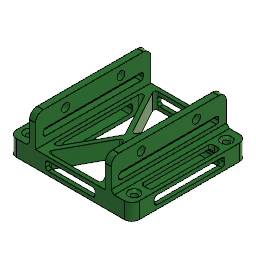
Full Motor Build (Goalie) (Autodesk Fusion 360 archive; units mm, degrees)
design "LGR Foundation"
Autodesk Fusion 360 part; units mm, degrees
(part 1 of 5)
sketch "Sketch1" plane through (0, 0, 0) normal (0, 0, 1) x (1, 0, 0)
  line L0 (-40, 37.5) -> (40, 37.5)
  line L1 (40, 37.5) -> (40, -37.5)
  line L2 (40, -37.5) -> (-40, -37.5)
  line L3 (-40, -37.5) -> (-40, 37.5)
  dimension "d1" = 80
  dimension "d2" = 75
  dimension "d3" = 37.5
  dimension "d4" = 40
  constraint horizontal L0
  constraint vertical L1
  constraint horizontal L2
  constraint vertical L3
  measures "d1" distance of L1 L3
  measures "d2" distance of L0 L2
  measures "d3" distance of origin L2
  measures "d4" distance of origin L1
extrude "Extrude1" add sketch "Sketch1" along normal blind 6
sketch "Sketch2" plane through (0, 0, 6) normal (0, 0, 1) x (-1, 0, 0)
  line L0 (40, 37.5) -> (-40, 37.5)
  line L1 (-40, 37.5) -> (-40, -37.5)
  line L2 (-40, -37.5) -> (40, -37.5)
  line L3 (40, -37.5) -> (40, 37.5)
  line L4 (26.55, -37.5) -> (22.55, -37.5)
  line L5 (22.55, -37.5) -> (22.55, 37.5)
  line L6 (22.55, 37.5) -> (26.55, 37.5)
  line L7 (26.55, 37.5) -> (26.55, -37.5)
  line L8 (-22.55, -37.5) -> (-26.55, -37.5)
  line L9 (-26.55, -37.5) -> (-26.55, 37.5)
  line L10 (-26.55, 37.5) -> (-22.55, 37.5)
  line L11 (-22.55, 37.5) -> (-22.55, -37.5)
  dimension "d7" = 45.1
  dimension "d8" = 53.1
  dimension "d9" = 13.45
  dimension "d10" = 17.45
  constraint horizontal L4
  constraint vertical L5
  constraint horizontal L6
  constraint vertical L7
  constraint coincident L0 L5.end
  constraint coincident L2 L4.start
  constraint horizontal L8
  constraint vertical L9
  constraint horizontal L10
  constraint vertical L11
  constraint coincident L0 L9.end
  constraint coincident L2 L8.start
  measures "d7" distance of L5 L11
  measures "d8" distance of L7 L9
  measures "d9" distance of L3 L7
  measures "d10" distance of L3 L5
extrude "Extrude2" add sketch "Sketch2" along normal blind 20 contours L0 L2 L4 L5 L6 L7 | L0 L2 L8 L9 L10 L11
sketch "Sketch3" plane through (26.55, 0, 0) normal (1, 0, 0) x (0, 1, 0)
  line L0 (-37.5, 6) -> (37.5, 6)
  line L1 (37.5, 6) -> (37.5, 26)
  line L2 (37.5, 26) -> (-37.5, 26)
  line L3 (-37.5, 26) -> (-37.5, 6)
  circle A0 centre (-18, 20) radius 2.55
  circle A1 centre (18, 20) radius 2.55
  line L4 (37.5, 0) -> (-37.5, 0)
  dimension "d13" = 5.1
  dimension "d14" = 5.1
  dimension "d15" = 20
  dimension "d16" = 36
  dimension "d17" = 19.5
  constraint horizontal A0.centre A1.centre
  measures "d13" diameter of A0
  measures "d14" diameter of A1
  measures "d15" distance of A0.centre L4
  measures "d16" distance of A0.centre A1.centre
  measures "d17" distance of L1 A1.centre
extrude "Extrude3" cut sketch "Sketch3" along normal blind 0 and the other way blind 53.1 contours A0 | A1
chamfer "Chamfer1" distance 2 angle 45 2 edges at (26.55, 0, 6) (-26.55, 0, 6)
sketch "Sketch8" plane through (0, 0, 6) normal (0, 0, 1) x (-1, 0, 0)
  line L0 (28.55, 37.5) -> (28.55, -37.5)
  line L1 (28.55, -37.5) -> (40, -37.5)
  line L2 (40, -37.5) -> (40, 37.5)
  line L3 (40, 37.5) -> (28.55, 37.5)
  line L4 (-40, 37.5) -> (-40, -37.5)
  line L5 (-40, -37.5) -> (-28.55, -37.5)
  point P0 (34, -30)
  point P1 (-34, -30)
  point P2 (-34, 30)
  point P3 (34, 30)
  dimension "d57" = 68
  dimension "d58" = 60
  dimension "d59" = 6
  dimension "d60" = 7.5
  constraint horizontal P0 P1
  constraint vertical P1 P2
  constraint horizontal P2 P3
  constraint vertical P0 P3
  measures "d57" distance of P0 P1
  measures "d58" distance of P1 P2
  measures "d59" distance of P1 L4
  measures "d60" distance of P1 L5
hole "Hole3" at (-34, 30, 6) at (-34, -30, 6) at (34, -30, 6) at (34, 30, 6) direction (0, 0, -1) diameter 3.797 end through all countersink diameter 7.087 countersink angle 100
fillet "Fillet1" radius 5 4 edges at (40, -37.5, 3) (40, 37.5, 3) (-40, -37.5, 3) (-40, 37.5, 3)
fillet "Fillet2" radius 5 4 edges at (24.55, -37.5, 26) (-24.55, -37.5, 26) (-24.55, 37.5, 26) (24.55, 37.5, 26)
sketch "Sketch13" plane through (0, 0, 6) normal (0, 0, 1) x (-1, 0, 0)
  line L0 (-22.55, 37.5) -> (-22.55, -37.5)
  line L1 (-22.55, -37.5) -> (22.55, -37.5)
  line L2 (22.55, -37.5) -> (22.55, 37.5)
  line L3 (22.55, 37.5) -> (-22.55, 37.5)
  line L4 (20.05, 27.1318) -> (20.05, -27.1318)
  line L5 (15.4698, 35) -> (-15.4698, 35)
  line L6 (-20.05, 27.1318) -> (-20.05, -27.1318)
  line L7 (15.4698, -35) -> (-15.4698, -35)
  line L8 (17.234, 27.8516) -> (2.3937, 0.7198)
  line L9 (2.3937, -0.7198) -> (17.234, -27.8516)
  line L10 (16.7858, -32.7802) -> (1.316, -4.4974)
  line L11 (-1.316, -4.4974) -> (-16.7858, -32.7802)
  line L12 (-17.234, -27.8516) -> (-2.3937, -0.7198)
  line L13 (-2.3937, 0.7198) -> (-17.234, 27.8516)
  line L14 (-16.7858, 32.7802) -> (-1.316, 4.4974)
  line L15 (1.316, 4.4974) -> (16.7858, 32.7802)
  arc A0 (20.05, 27.1318) -> (17.234, 27.8516) centre (18.55, 27.1318) ccw
  arc A1 (17.234, -27.8516) -> (20.05, -27.1318) centre (18.55, -27.1318) ccw
  arc A2 (15.4698, -35) -> (16.7858, -32.7802) centre (15.4698, -33.5) ccw
  arc A3 (16.7858, 32.7802) -> (15.4698, 35) centre (15.4698, 33.5) ccw
  arc A4 (-15.4698, 35) -> (-16.7858, 32.7802) centre (-15.4698, 33.5) ccw
  arc A5 (-17.234, 27.8516) -> (-20.05, 27.1318) centre (-18.55, 27.1318) ccw
  arc A6 (-20.05, -27.1318) -> (-17.234, -27.8516) centre (-18.55, -27.1318) ccw
  arc A7 (-16.7858, -32.7802) -> (-15.4698, -35) centre (-15.4698, -33.5) ccw
  arc A8 (1.316, -4.4974) -> (-1.316, -4.4974) centre (0, -5.2172) ccw
  arc A9 (2.3937, 0.7198) -> (2.3937, -0.7198) centre (3.7097, 0) ccw
  arc A10 (-1.316, 4.4974) -> (1.316, 4.4974) centre (0, 5.2172) ccw
  arc A11 (-2.3937, -0.7198) -> (-2.3937, 0.7198) centre (-3.7097, 0) ccw
  point P0 (20.05, 33)
  point P1 (20.05, -33)
  point P2 (18, 35)
  point P3 (-18, 35)
  point P4 (-20.05, 33)
  point P5 (-20.05, -33)
  point P6 (18, -35)
  point P7 (-18, -35)
  dimension "d91" = 2.5
  dimension "d92" = 2.5
  dimension "d93" = 66
  dimension "d95" = 66
  dimension "d96" = 2.5
  dimension "d97" = 36
  dimension "d98" = 36
  dimension "d99" = 2.5
  dimension "d100" = 4.55
  dimension "d101" = 4.55
  dimension "d102" = 4.5
  dimension "d103" = 4.5
  dimension "d104" = 1.5
  constraint vertical L4
  constraint horizontal L5
  constraint parallel L0 L6
  constraint horizontal L7
  constraint parallel L9 L10
  constraint parallel L8 L11
  constraint parallel L11 L12
  constraint parallel L13 L14
  constraint coincident P0 L4
  constraint coincident P0 L8
  constraint tangent L4 A0
  constraint tangent L8 A0
  constraint coincident P1 L4
  constraint coincident P1 L9
  constraint tangent L4 A1
  constraint tangent L9 A1
  constraint equal A0 A1
  constraint coincident P6 L10
  constraint coincident P6 L7
  constraint tangent L10 A2
  constraint tangent L7 A2
  constraint equal A0 A2
  constraint coincident P2 L15
  constraint coincident P2 L5
  constraint tangent L15 A3
  constraint tangent L5 A3
  constraint equal A0 A3
  constraint coincident P3 L14
  constraint coincident P3 L5
  constraint tangent L14 A4
  constraint tangent L5 A4
  constraint equal A0 A4
  constraint coincident P4 L13
  constraint coincident P4 L6
  constraint tangent L13 A5
  constraint tangent L6 A5
  constraint equal A0 A5
  constraint coincident P5 L6
  constraint coincident P5 L12
  constraint tangent L6 A6
  constraint tangent L12 A6
  constraint equal A0 A6
  constraint coincident P7 L11
  constraint coincident P7 L7
  constraint tangent L11 A7
  constraint tangent L7 A7
  constraint equal A0 A7
  constraint tangent L10 A8
  constraint tangent L11 A8
  constraint equal A0 A8
  constraint tangent L9 A9
  constraint tangent L8 A9
  constraint equal A0 A9
  constraint tangent L15 A10
  constraint tangent L14 A10
  constraint equal A0 A10
  constraint tangent L13 A11
  constraint tangent L12 A11
  constraint equal A0 A11
  measures "d91" distance of L2 L4
  measures "d92" distance of L3 L5
  measures "d93" distance of P0 P1
  measures "d95" distance of P4 P5
  measures "d96" distance of L0 L6
  measures "d97" distance of P6 P7
  measures "d98" distance of P2 P3
  measures "d99" distance of L1 L7
  measures "d100" distance of L2 P6
  measures "d101" distance of L2 P2
  measures "d102" distance of L3 P0
  measures "d103" distance of L3 P4
  measures "d104" radius of A0
extrude "Extrude6" cut sketch "Sketch13" along normal blind 0 and the other way blind 6 contours L4 L8 L9 A0 A1 A9 | L5 L14 L15 A3 A4 A10 | L6 L12 L13 A5 A6 A11 | L7 L10 L11 A2 A7 A8
extrude "Extrude7" cut 1 faces at (29.1614, 9.0439, 0) along direction (0, 0, -1) blind 0 and the other way blind 0.4
ref_plane "WorkPlane3" through (34.275, 0, 1.9) normal (0, 0, 1) x (1, 0, 0)
sketch "Sketch14" plane through (0, 0, 1.9) normal (0, 0, 1) x (1, 0, 0)
  circle A0 centre (34, 30) radius 4.5
  circle A1 centre (-34, 30) radius 4.5
  circle A2 centre (-34, -30) radius 4.5
  circle A3 centre (34, -30) radius 4.5
  line L0 (35, 37.5) -> (28.55, 37.5)
  line L1 (40, -32.5) -> (40, 32.5)
  dimension "d115" = 9
  dimension "d116" = 9
  dimension "d117" = 9
  dimension "d118" = 9
  dimension "d119" = 68
  dimension "d120" = 60
  dimension "d121" = 7.5
  dimension "d122" = 6
  constraint horizontal A0.centre A1.centre
  constraint vertical A0.centre A3.centre
  constraint horizontal A2.centre A3.centre
  constraint vertical A1.centre A2.centre
  measures "d115" diameter of A0
  measures "d116" diameter of A1
  measures "d117" diameter of A2
  measures "d118" diameter of A3
  measures "d119" distance of A0.centre A1.centre
  measures "d120" distance of A0.centre A3.centre
  measures "d121" distance of A0.centre L0
  measures "d122" distance of A0.centre L1
ref_plane "WorkPlane4" through (34.275, 0, 0.4) normal (0, 0, 1) x (1, 0, 0)
sketch "Sketch17" plane through (0, 0, 6) normal (0, 0, 1) x (-1, 0, 0)
  arc A0 (-40, -32.5) -> (-35, -37.5) centre (-35, -32.5) ccw
  line L0 (-35, -37.5) -> (-28.55, -37.5)
  line L1 (-28.55, -37.5) -> (-28.55, 37.5)
  line L2 (-28.55, 37.5) -> (-35, 37.5)
  arc A1 (-35, 37.5) -> (-40, 32.5) centre (-35, 32.5) ccw
  line L3 (-40, 32.5) -> (-40, -32.5)
  line L4 (-33.05, -23) -> (-35.5, -23)
  line L5 (-37.5, -21) -> (-37.5, 21)
  line L6 (-35.5, 23) -> (-33.05, 23)
  line L7 (-31.05, 21) -> (-31.05, -21)
  arc A2 (-33.05, -23) -> (-31.05, -21) centre (-33.05, -21) ccw
  arc A3 (-31.05, 21) -> (-33.05, 23) centre (-33.05, 21) ccw
  arc A4 (-35.5, 23) -> (-37.5, 21) centre (-35.5, 21) ccw
  arc A5 (-37.5, -21) -> (-35.5, -23) centre (-35.5, -21) ccw
  line L8 (35.5, -23) -> (33.05, -23)
  line L9 (31.05, -21) -> (31.05, 21)
  line L10 (33.05, 23) -> (35.5, 23)
  line L11 (37.5, 21) -> (37.5, -21)
  line L12 (28.55, -37.5) -> (28.55, 37.5)
  line L13 (40, -32.5) -> (40, 32.5)
  arc A6 (35.5, -23) -> (37.5, -21) centre (35.5, -21) ccw
  arc A7 (31.05, -21) -> (33.05, -23) centre (33.05, -21) ccw
  arc A8 (33.05, 23) -> (31.05, 21) centre (33.05, 21) ccw
  arc A9 (37.5, 21) -> (35.5, 23) centre (35.5, 21) ccw
  circle A10 centre (-34, 30) radius 3.5435
  circle A11 centre (-34, -30) radius 3.5435
  point P0 (-34, -30)
  point P1 (-34, 30)
  point P2 (34, -30)
  point P3 (34, 30)
  dimension "d134" = 2.5
  dimension "d135" = 2.5
  dimension "d136" = 7
  dimension "d137" = 7
  dimension "d138" = 2
  dimension "d141" = 2.5
  dimension "d142" = 2.5
  dimension "d143" = 7
  dimension "d144" = 7
  dimension "d145" = 2
  constraint horizontal L4
  constraint vertical L5
  constraint horizontal L6
  constraint vertical L7
  constraint tangent L4 A2
  constraint tangent L7 A2
  constraint tangent L6 A3
  constraint tangent L7 A3
  constraint equal A2 A3
  constraint tangent L6 A4
  constraint tangent L5 A4
  constraint equal A2 A4
  constraint tangent L5 A5
  constraint tangent L4 A5
  constraint equal A2 A5
  constraint horizontal L8
  constraint vertical L9
  constraint horizontal L10
  constraint vertical L11
  constraint tangent L8 A6
  constraint tangent L11 A6
  constraint tangent L9 A7
  constraint tangent L8 A7
  constraint equal A6 A7
  constraint tangent L9 A8
  constraint tangent L10 A8
  constraint equal A6 A8
  constraint tangent L10 A9
  constraint tangent L11 A9
  constraint equal A6 A9
  measures "d134" distance of L1 L7
  measures "d135" distance of L3 L5
  measures "d136" distance of L4 P0
  measures "d137" distance of L6 P1
  measures "d138" radius of A2
  measures "d141" distance of L9 L12
  measures "d142" distance of L11 L13
  measures "d143" distance of L8 P2
  measures "d144" distance of L10 P3
  measures "d145" radius of A6
extrude "Extrude10" cut sketch "Sketch17" against normal blind 5.6 contours L4 L5 L6 L7 A2 A3 A4 A5 | L8 L9 L10 L11 A6 A7 A8 A9
extrude "Extrude12" add 1 faces at (-23.7167, 7, 0.4) along direction (0, 0, -1) blind 5
sketch "Sketch18" plane through (0, -37.5, 0) normal (0, -1, 0) x (1, 0, 0)
  line L0 (35, -4.6) -> (35, 6)
  line L1 (35, 6) -> (28.55, 6)
  line L2 (28.55, 6) -> (26.55, 8)
  line L3 (26.55, 8) -> (26.55, 21)
  line L4 (26.55, 21) -> (22.55, 21)
  line L5 (22.55, 21) -> (22.55, 6)
  line L6 (22.55, 6) -> (-22.55, 6)
  line L7 (-22.55, 6) -> (-22.55, 21)
  line L8 (-22.55, 21) -> (-26.55, 21)
  line L9 (-26.55, 21) -> (-26.55, 8)
  line L10 (-26.55, 8) -> (-28.55, 6)
  line L11 (-28.55, 6) -> (-35, 6)
  line L12 (-35, 6) -> (-35, -4.6)
  line L13 (-35, -4.6) -> (35, -4.6)
  line L14 (-14.5, 3.5) -> (14.5, 3.5)
  line L15 (16, 2) -> (16, -0.6)
  line L16 (14.5, -2.1) -> (-14.5, -2.1)
  line L17 (-16, -0.6) -> (-16, 2)
  arc A0 (-14.5, 3.5) -> (-16, 2) centre (-14.5, 2) ccw
  arc A1 (-16, -0.6) -> (-14.5, -2.1) centre (-14.5, -0.6) ccw
  arc A2 (14.5, -2.1) -> (16, -0.6) centre (14.5, -0.6) ccw
  arc A3 (16, 2) -> (14.5, 3.5) centre (14.5, 2) ccw
  dimension "d154" = 32
  dimension "d155" = 2.5
  dimension "d156" = 2.5
  dimension "d157" = 16
  dimension "d158" = 1.5
  constraint horizontal L14
  constraint vertical L15
  constraint horizontal L16
  constraint vertical L17
  constraint tangent L14 A0
  constraint tangent L17 A0
  constraint tangent L17 A1
  constraint tangent L16 A1
  constraint equal A0 A1
  constraint tangent L16 A2
  constraint tangent L15 A2
  constraint equal A0 A2
  constraint tangent L15 A3
  constraint tangent L14 A3
  constraint equal A0 A3
  measures "d154" distance of L15 L17
  measures "d155" distance of L6 L14
  measures "d156" distance of L13 L16
  measures "d157" distance of origin L17
  measures "d158" radius of A0
extrude "Extrude13" cut sketch "Sketch18" against normal blind 4 contours L14 L15 L16 L17 A0 A1 A2 A3
sketch "Sketch19" plane through (0, 37.5, 0) normal (0, 1, 0) x (-1, 0, 0)
  line L0 (35, -4.6) -> (35, 6)
  line L1 (35, 6) -> (28.55, 6)
  line L2 (28.55, 6) -> (26.55, 8)
  line L3 (26.55, 8) -> (26.55, 21)
  line L4 (26.55, 21) -> (22.55, 21)
  line L5 (22.55, 21) -> (22.55, 6)
  line L6 (22.55, 6) -> (-22.55, 6)
  line L7 (-22.55, 6) -> (-22.55, 21)
  line L8 (-22.55, 21) -> (-26.55, 21)
  line L9 (-26.55, 21) -> (-26.55, 8)
  line L10 (-26.55, 8) -> (-28.55, 6)
  line L11 (-28.55, 6) -> (-35, 6)
  line L12 (-35, 6) -> (-35, -4.6)
  line L13 (-35, -4.6) -> (35, -4.6)
  line L14 (-14.5, 3.5) -> (14.5, 3.5)
  line L15 (16, 2) -> (16, -0.6)
  line L16 (14.5, -2.1) -> (-14.5, -2.1)
  line L17 (-16, -0.6) -> (-16, 2)
  arc A0 (-14.5, 3.5) -> (-16, 2) centre (-14.5, 2) ccw
  arc A1 (-16, -0.6) -> (-14.5, -2.1) centre (-14.5, -0.6) ccw
  arc A2 (14.5, -2.1) -> (16, -0.6) centre (14.5, -0.6) ccw
  arc A3 (16, 2) -> (14.5, 3.5) centre (14.5, 2) ccw
  dimension "d161" = 2.5
  dimension "d162" = 2.5
  dimension "d163" = 32
  dimension "d164" = 16
  dimension "d165" = 1.5
  constraint horizontal L14
  constraint vertical L15
  constraint horizontal L16
  constraint vertical L17
  constraint tangent L14 A0
  constraint tangent L17 A0
  constraint tangent L17 A1
  constraint tangent L16 A1
  constraint equal A0 A1
  constraint tangent L16 A2
  constraint tangent L15 A2
  constraint equal A0 A2
  constraint tangent L15 A3
  constraint tangent L14 A3
  constraint equal A0 A3
  measures "d161" distance of L13 L16
  measures "d162" distance of L6 L14
  measures "d163" distance of L15 L17
  measures "d164" distance of origin L17
  measures "d165" radius of A0
extrude "Extrude14" cut sketch "Sketch19" against normal blind 4 contours L14 L15 L16 L17 A0 A1 A2 A3
sketch "Sketch20" plane through (-40, 0, 0) normal (-1, 0, 0) x (0, -1, 0)
  line L0 (32.5, -4.6) -> (32.5, 6)
  line L1 (32.5, 6) -> (-32.5, 6)
  line L2 (-32.5, 6) -> (-32.5, -4.6)
  line L3 (-32.5, -4.6) -> (32.5, -4.6)
  line L4 (-21, 3.5) -> (21, 3.5)
  line L5 (23, 1.5) -> (23, -0.1)
  line L6 (21, -2.1) -> (-21, -2.1)
  line L7 (-23, -0.1) -> (-23, 1.5)
  line L8 (-32.5, 6) -> (32.5, 6)
  arc A0 (-21, 3.5) -> (-23, 1.5) centre (-21, 1.5) ccw
  arc A1 (-23, -0.1) -> (-21, -2.1) centre (-21, -0.1) ccw
  arc A2 (21, -2.1) -> (23, -0.1) centre (21, -0.1) ccw
  arc A3 (23, 1.5) -> (21, 3.5) centre (21, 1.5) ccw
  dimension "d168" = 2.5
  dimension "d169" = 2.5
  dimension "d170" = 46
  dimension "d171" = 23
  dimension "d172" = 2
  constraint horizontal L4
  constraint vertical L5
  constraint horizontal L6
  constraint vertical L7
  constraint tangent L4 A0
  constraint tangent L7 A0
  constraint tangent L7 A1
  constraint tangent L6 A1
  constraint equal A0 A1
  constraint tangent L6 A2
  constraint tangent L5 A2
  constraint equal A0 A2
  constraint tangent L5 A3
  constraint tangent L4 A3
  constraint equal A0 A3
  measures "d168" distance of L4 L8
  measures "d169" distance of L3 L6
  measures "d170" distance of L5 L7
  measures "d171" distance of origin L7
  measures "d172" radius of A0
extrude "Extrude15" cut sketch "Sketch20" against normal blind 22 contours L4 L5 L6 L7 A0 A1 A2 A3
sketch "Sketch21" plane through (40, 0, 0) normal (1, 0, 0) x (0, 1, 0)
  line L0 (32.5, -4.6) -> (32.5, 6)
  line L1 (32.5, 6) -> (-32.5, 6)
  line L2 (-32.5, 6) -> (-32.5, -4.6)
  line L3 (-32.5, -4.6) -> (32.5, -4.6)
  line L4 (-21, 3.5) -> (21, 3.5)
  line L5 (23, 1.5) -> (23, -0.1)
  line L6 (21, -2.1) -> (-21, -2.1)
  line L7 (-23, -0.1) -> (-23, 1.5)
  line L8 (21, 6) -> (-21, 6)
  arc A0 (-21, 3.5) -> (-23, 1.5) centre (-21, 1.5) ccw
  arc A1 (-23, -0.1) -> (-21, -2.1) centre (-21, -0.1) ccw
  arc A2 (21, -2.1) -> (23, -0.1) centre (21, -0.1) ccw
  arc A3 (23, 1.5) -> (21, 3.5) centre (21, 1.5) ccw
  dimension "d175" = 2.5
  dimension "d176" = 2.5
  dimension "d177" = 46
  dimension "d178" = 23
  dimension "d179" = 2
  constraint horizontal L4
  constraint vertical L5
  constraint horizontal L6
  constraint vertical L7
  constraint tangent L4 A0
  constraint tangent L7 A0
  constraint tangent L7 A1
  constraint tangent L6 A1
  constraint equal A0 A1
  constraint tangent L6 A2
  constraint tangent L5 A2
  constraint equal A0 A2
  constraint tangent L5 A3
  constraint tangent L4 A3
  constraint equal A0 A3
  measures "d175" distance of L4 L8
  measures "d176" distance of L3 L6
  measures "d177" distance of L5 L7
  measures "d178" distance of origin L5
  measures "d179" radius of A0
extrude "Extrude16" cut sketch "Sketch21" against normal blind 22 contours L4 L5 L6 L7 A0 A1 A2 A3
sketch "Sketch23" plane through (26.55, 0, 0) normal (1, 0, 0) x (0, 1, 0)
  arc A0 (37.5, 21) -> (32.5, 26) centre (32.5, 21) ccw
  line L0 (32.5, 26) -> (-32.5, 26)
  arc A1 (-32.5, 26) -> (-37.5, 21) centre (-32.5, 21) ccw
  line L1 (-37.5, 21) -> (-37.5, 8)
  line L2 (-37.5, 8) -> (37.5, 8)
  line L3 (37.5, 8) -> (37.5, 21)
  circle A2 centre (-18, 20) radius 2.55
  circle A3 centre (18, 20) radius 2.55
  line L4 (-31, 14.95) -> (31, 14.95)
  line L5 (32.5, 13.45) -> (32.5, 12)
  line L6 (31, 10.5) -> (-31, 10.5)
  line L7 (-32.5, 12) -> (-32.5, 13.45)
  arc A4 (-31, 14.95) -> (-32.5, 13.45) centre (-31, 13.45) ccw
  arc A5 (-32.5, 12) -> (-31, 10.5) centre (-31, 12) ccw
  arc A6 (31, 10.5) -> (32.5, 12) centre (31, 12) ccw
  arc A7 (32.5, 13.45) -> (31, 14.95) centre (31, 13.45) ccw
  dimension "d186" = 2.5
  dimension "d187" = 5
  dimension "d188" = 5
  dimension "d189" = 5.05
  dimension "d190" = 1.5
  constraint horizontal L4
  constraint vertical L5
  constraint horizontal L6
  constraint vertical L7
  constraint tangent L4 A4
  constraint tangent L7 A4
  constraint tangent L7 A5
  constraint tangent L6 A5
  constraint equal A4 A5
  constraint tangent L6 A6
  constraint tangent L5 A6
  constraint equal A4 A6
  constraint tangent L5 A7
  constraint tangent L4 A7
  constraint equal A4 A7
  measures "d186" distance of L2 L6
  measures "d187" distance of L1 L7
  measures "d188" distance of L3 L5
  measures "d189" distance of A2.centre L4
  measures "d190" radius of A4
extrude "Extrude17" cut sketch "Sketch23" against normal blind 55 contours L4 L5 L6 L7 A4 A5 A6 A7
equation "d3 = ( 75 / 2 ) * 1 mm"
equation "d4 = ( 80 / 2 ) * 1 mm"
equation "d9 = ( ( 80 - 53.1 ) / 2 ) * 1 mm"
equation "d10 = ( ( 80 - 45.1 ) / 2 ) * 1 mm"
equation "d17 = ( ( 75 - 36 ) / 2 ) * 1 mm"
equation "d59 = ( ( 80 - 68 ) / 2 ) * 1 mm"
equation "d60 = ( ( 75 - 60 ) / 2 ) * 1 mm"
equation "d100 = ( ( 45.1 - 36 ) / 2 ) * 1 mm"
equation "d101 = ( ( 45.1 - 36 ) / 2 ) * 1 mm"
equation "d102 = ( ( 75 - 66 ) / 2 ) * 1 mm"
equation "d103 = ( ( 75 - 66 ) / 2 ) * 1 mm"
equation "d171 = ( 46 / 2 ) * 1 mm"
equation "d189 = ( ( 5.1 / 2 ) * 1 mm ) + 2.5 mm"

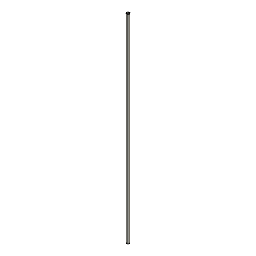
design "Foosball Rod"
Autodesk Fusion 360 part; units mm, degrees
sketch "Sketch1" plane through (0, 0, 0) normal (0, 0, 1) x (1, 0, 0)
  circle A0 centre (0, 0) radius 7.9375
  circle A1 centre (0, 0) radius 6.35
  dimension "d1" = 15.875
  dimension "d2" = 12.7
  constraint coincident A0.centre A1.centre
  constraint concentric A0 A1
  measures "d1" diameter of A0
  measures "d2" diameter of A1
extrude "Extrude1" add sketch "Sketch1" along normal blind 1130.3
equation "d1 = 0'- 5/8\""
equation "d2 = 0'- 1/2\""

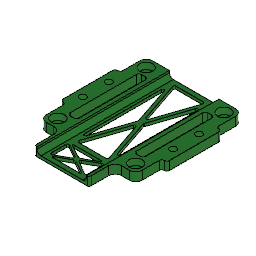
design "LGR RM Carriage Bracket (Goalie)"
Autodesk Fusion 360 part; units mm, degrees
sketch "Sketch1" plane through (0, 0, 0) normal (0, 0, 1) x (1, 0, 0)
  line L0 (-41, 41) -> (41, 41)
  line L1 (41, 41) -> (41, -41)
  line L2 (41, -41) -> (-41, -41)
  line L3 (-41, -41) -> (-41, 41)
  dimension "d1" = 82
  dimension "d2" = 82
  dimension "d3" = 41
  dimension "d4" = 41
  constraint horizontal L0
  constraint vertical L1
  constraint horizontal L2
  constraint vertical L3
  measures "d1" distance of L1 L3
  measures "d2" distance of L0 L2
  measures "d3" distance of origin L1
  measures "d4" distance of origin L0
extrude "Extrude1" add sketch "Sketch1" along normal blind 6.5
sketch "Sketch2" plane through (0, 0, 6.5) normal (0, 0, 1) x (-1, 0, 0)
  line L0 (41, 41) -> (-41, 41)
  line L1 (-41, 41) -> (-41, -41)
  line L2 (-41, -41) -> (41, -41)
  line L3 (41, -41) -> (41, 41)
  point P0 (34, -30)
  point P1 (-34, -30)
  point P2 (-34, 30)
  point P3 (34, 30)
  dimension "d7" = 68
  dimension "d8" = 60
  dimension "d9" = 7
  dimension "d10" = 11
  constraint horizontal P0 P1
  constraint vertical P1 P2
  constraint horizontal P2 P3
  constraint vertical P0 P3
  measures "d7" distance of P0 P1
  measures "d8" distance of P1 P2
  measures "d9" distance of L1 P1
  measures "d10" distance of L2 P1
hole "Hole1" at (-34, 30, 6.5) at (34, 30, 6.5) at (34, -30, 6.5) at (-34, -30, 6.5) direction (0, 0, -1) diameter 5.5 depth 10 tip angle 180 counterbore diameter 10 counterbore depth 5
sketch "Sketch3" plane through (0, 0, 6.5) normal (0, 0, 1) x (-1, 0, 0)
  circle A0 centre (-34, 30) radius 5
  circle A1 centre (34, -30) radius 5
  circle A2 centre (-34, -30) radius 5
  circle A3 centre (34, 30) radius 5
  line L0 (41, 41) -> (-41, 41)
  line L1 (-41, 41) -> (-41, -41)
  line L2 (-41, -41) -> (41, -41)
  line L3 (41, -41) -> (41, 41)
  line L4 (41, -19.05) -> (-41, -19.05)
  line L5 (-41, -19.05) -> (-41, 19.05)
  line L6 (-41, 19.05) -> (41, 19.05)
  line L7 (41, 19.05) -> (41, -19.05)
  dimension "d16" = 38.1
  dimension "d17" = 19.05
  constraint horizontal L4
  constraint vertical L5
  constraint horizontal L6
  constraint vertical L7
  constraint coincident L1 L5.end
  constraint coincident L3 L4.start
  measures "d16" distance of L4 L6
  measures "d17" distance of origin L6
extrude "Extrude2" cut sketch "Sketch3" against normal blind 4.5 contours L1 L3 L4 L5 L6 L7
fillet "Fillet1" radius 3 2 edges at (0, 19.05, 2) (0, -19.05, 2)
sketch "Sketch4" plane through (0, 0, 6.5) normal (0, 0, 1) x (-1, 0, 0)
  line L0 (41, -19.05) -> (-41, -19.05)
  line L1 (-41, -19.05) -> (-41, -41)
  line L2 (-41, -41) -> (41, -41)
  line L3 (41, -41) -> (41, -19.05)
  circle A0 centre (34, -30) radius 5
  circle A1 centre (-34, -30) radius 5
  line L4 (41, 41) -> (-41, 41)
  line L5 (41, 19.05) -> (41, 41)
  point P0 (-10, -34.75)
  point P1 (10, -34.75)
  point P2 (-10, 34.75)
  point P3 (10, 34.75)
  point P4 (-5.7919, 53.9874)
  dimension "d23" = 6.25
  dimension "d24" = 6.25
  dimension "d25" = 20
  dimension "d26" = 31
  constraint vertical P0 P2
  constraint horizontal P2 P3
  constraint vertical P1 P3
  constraint horizontal P0 P1
  measures "d23" distance of P2 L4
  measures "d24" distance of L2 P0
  measures "d25" distance of P0 P1
  measures "d26" distance of P3 L5
hole "Hole2" at (10, 34.75, 6.5) at (-10, 34.75, 6.5) at (10, -34.75, 6.5) at (-10, -34.75, 6.5) direction (0, 0, -1) diameter 5 end through all
sketch "Sketch7" plane through (0, 0, 6.5) normal (0, 0, 1) x (-1, 0, 0)
  circle A0 centre (-10, 34.75) radius 2.5
  circle A1 centre (10, 34.75) radius 2.5
  line L0 (-41, 19.05) -> (41, 19.05)
  line L1 (41, 19.05) -> (41, 41)
  line L2 (41, 41) -> (-41, 41)
  line L3 (-41, 41) -> (-41, 19.05)
  circle A2 centre (34, 30) radius 5
  circle A3 centre (-34, 30) radius 5
  line L4 (25.5, 22.05) -> (-25.5, 22.05)
  line L5 (-27.5, 24.05) -> (-27.5, 27.05)
  line L6 (-25.5, 29.05) -> (25.5, 29.05)
  line L7 (27.5, 27.05) -> (27.5, 24.05)
  line L8 (25.5, -29.05) -> (-25.5, -29.05)
  line L9 (-27.5, -27.05) -> (-27.5, -24.05)
  line L10 (-25.5, -22.05) -> (25.5, -22.05)
  line L11 (27.5, -24.05) -> (27.5, -27.05)
  line L12 (41, -19.05) -> (-41, -19.05)
  line L13 (-41, -19.05) -> (-41, -41)
  arc A4 (25.5, -29.05) -> (27.5, -27.05) centre (25.5, -27.05) ccw
  arc A5 (27.5, -24.05) -> (25.5, -22.05) centre (25.5, -24.05) ccw
  arc A6 (-25.5, -22.05) -> (-27.5, -24.05) centre (-25.5, -24.05) ccw
  arc A7 (-27.5, -27.05) -> (-25.5, -29.05) centre (-25.5, -27.05) ccw
  arc A8 (25.5, 22.05) -> (27.5, 24.05) centre (25.5, 24.05) ccw
  arc A9 (27.5, 27.05) -> (25.5, 29.05) centre (25.5, 27.05) ccw
  arc A10 (-25.5, 29.05) -> (-27.5, 27.05) centre (-25.5, 27.05) ccw
  arc A11 (-27.5, 24.05) -> (-25.5, 22.05) centre (-25.5, 24.05) ccw
  dimension "d31" = 55
  dimension "d32" = 7
  dimension "d33" = 3
  dimension "d34" = 13.5
  dimension "d35" = 7
  dimension "d36" = 3
  dimension "d37" = 13.5
  dimension "d38" = 55
  dimension "d39" = 2
  constraint horizontal L4
  constraint vertical L5
  constraint horizontal L6
  constraint vertical L7
  constraint horizontal L8
  constraint vertical L9
  constraint horizontal L10
  constraint vertical L11
  constraint tangent L8 A4
  constraint tangent L11 A4
  constraint tangent L11 A5
  constraint tangent L10 A5
  constraint equal A4 A5
  constraint tangent L10 A6
  constraint tangent L9 A6
  constraint equal A4 A6
  constraint tangent L9 A7
  constraint tangent L8 A7
  constraint equal A4 A7
  constraint tangent L4 A8
  constraint tangent L7 A8
  constraint equal A4 A8
  constraint tangent L7 A9
  constraint tangent L6 A9
  constraint equal A4 A9
  constraint tangent L6 A10
  constraint tangent L5 A10
  constraint equal A4 A10
  constraint tangent L5 A11
  constraint tangent L4 A11
  constraint equal A4 A11
  measures "d31" distance of L5 L7
  measures "d32" distance of L4 L6
  measures "d33" distance of L0 L4
  measures "d34" distance of L1 L7
  measures "d35" distance of L8 L10
  measures "d36" distance of L10 L12
  measures "d37" distance of L9 L13
  measures "d38" distance of L9 L11
  measures "d39" radius of A4
extrude "Extrude3" cut sketch "Sketch7" against normal blind 6.5 contours L4 L5 L6 L7 A8 A9 A10 A11 | L8 L9 L10 L11 A4 A5 A6 A7
ref_plane "WorkPlane1" through (0, 0, 6.5) normal (0, 0, -1) x (-1, 0, 0)
sketch "Sketch9" plane through (0, 0, 6.5) normal (0, 0, -1) x (-1, 0, 0)
  line L0 (41, 41) -> (21, 41)
  line L1 (21, 41) -> (21, 37)
  line L2 (21, 37) -> (41, 37)
  line L3 (41, 37) -> (41, 41)
  line L4 (-21, 41) -> (-41, 41)
  line L5 (-41, 41) -> (-41, 37)
  line L6 (-41, 37) -> (-21, 37)
  line L7 (-21, 37) -> (-21, 41)
  line L8 (41, -37) -> (21, -37)
  line L9 (21, -37) -> (21, -41)
  line L10 (21, -41) -> (41, -41)
  line L11 (41, -41) -> (41, -37)
  line L12 (-41, -41) -> (-21, -41)
  line L13 (-21, -41) -> (-21, -37)
  line L14 (-21, -37) -> (-41, -37)
  line L15 (-41, -37) -> (-41, -41)
  point P0 (41, 41)
  dimension "d59" = 82
  dimension "d60" = 82
  dimension "d61" = 4
  dimension "d62" = 20
  dimension "d63" = 20
  dimension "d64" = 4
  dimension "d65" = 20
  dimension "d66" = 20
  dimension "d67" = 4
  dimension "d68" = 4
  constraint horizontal L0
  constraint vertical L1
  constraint horizontal L2
  constraint vertical L3
  constraint horizontal L4
  constraint vertical L5
  constraint horizontal L6
  constraint vertical L7
  constraint horizontal L8
  constraint vertical L9
  constraint horizontal L10
  constraint vertical L11
  constraint horizontal L12
  constraint vertical L13
  constraint horizontal L14
  constraint vertical L15
  constraint vertical P0 L10.end
  constraint horizontal P0 L4.end
  constraint vertical L4.end L12.start
  constraint horizontal L10.end L12.start
  constraint vertical P0 L0.start
  constraint horizontal L0.end P0
  measures "d59" distance of L3 L5
  measures "d60" distance of L0 L10
  measures "d61" distance of L0 L2
  measures "d62" distance of L1 L3
  measures "d63" distance of L5 L7
  measures "d64" distance of L4 L6
  measures "d65" distance of L13 L15
  measures "d66" distance of L9 L11
  measures "d67" distance of L8 L10
  measures "d68" distance of L12 L14
extrude "Extrude5" cut sketch "Sketch9" along normal blind 6.5
fillet "Fillet2" radius 5 4 edges at (-41, 37, 3.25) (41, 37, 3.25) (41, -37, 3.25) (-41, -37, 3.25)
fillet "Fillet3" radius 2 8 edges at (-21, -41, 3.25) (-21, -37, 3.25) (21, -37, 3.25) (21, -41, 3.25) (21, 37, 3.25) (21, 41, 3.25) (-21, 41, 3.25) (-21, 37, 3.25)
sketch "Sketch10" plane through (0, 0, 2) normal (0, 0, 1) x (-1, 0, 0)
  line L0 (41, 16.05) -> (-41, 16.05)
  line L1 (-41, 16.05) -> (-41, -16.05)
  line L2 (-41, -16.05) -> (41, -16.05)
  line L3 (41, -16.05) -> (41, 16.05)
  line L4 (29.8377, -14) -> (-29.8377, -14)
  line L5 (29.8377, 14) -> (-29.8377, 14)
  line L6 (37.5, -10.6064) -> (37.5, 10.6064)
  line L7 (-37.5, -10.6064) -> (-37.5, 10.6064)
  line L8 (41, -19.05) -> (-41, -19.05)
  line L9 (30.154, 12.0513) -> (0.3162, 2.1054)
  line L10 (-0.3162, 2.1054) -> (-30.154, 12.0513)
  line L11 (-36.1798, 11.5537) -> (-4.8025, 0.9473)
  line L12 (-4.8025, -0.9473) -> (-36.1798, -11.5537)
  line L13 (-30.154, -12.0513) -> (-0.3162, -2.1054)
  line L14 (0.3162, -2.1054) -> (30.154, -12.0513)
  line L15 (36.1798, -11.5537) -> (4.8025, -0.9473)
  line L16 (4.8025, 0.9473) -> (36.1798, 11.5537)
  arc A0 (29.8377, -14) -> (30.154, -12.0513) centre (29.8377, -13) ccw
  arc A1 (0.3162, -2.1054) -> (-0.3162, -2.1054) centre (0, -3.0541) ccw
  arc A2 (-30.154, -12.0513) -> (-29.8377, -14) centre (-29.8377, -13) ccw
  arc A3 (-37.5, -10.6064) -> (-36.1798, -11.5537) centre (-36.5, -10.6064) ccw
  arc A4 (-36.1798, 11.5537) -> (-37.5, 10.6064) centre (-36.5, 10.6064) ccw
  arc A5 (-4.8025, -0.9473) -> (-4.8025, 0.9473) centre (-5.1228, 0) ccw
  arc A6 (-0.3162, 2.1054) -> (0.3162, 2.1054) centre (0, 3.0541) ccw
  arc A7 (-29.8377, 14) -> (-30.154, 12.0513) centre (-29.8377, 13) ccw
  arc A8 (30.154, 12.0513) -> (29.8377, 14) centre (29.8377, 13) ccw
  arc A9 (37.5, 10.6064) -> (36.1798, 11.5537) centre (36.5, 10.6064) ccw
  arc A10 (36.1798, -11.5537) -> (37.5, -10.6064) centre (36.5, -10.6064) ccw
  arc A11 (4.8025, 0.9473) -> (4.8025, -0.9473) centre (5.1228, 0) ccw
  point P0 (36, -14)
  point P1 (-36, -14)
  point P2 (-37.5, -12)
  point P3 (-37.5, 12)
  point P4 (0, -2)
  point P5 (-2, 0)
  point P6 (0, 2)
  point P7 (2, 0)
  dimension "d75" = 72
  dimension "d76" = 24
  dimension "d77" = 5
  dimension "d78" = 7.05
  dimension "d79" = 2.05
  dimension "d80" = 2.05
  dimension "d81" = 3.5
  dimension "d82" = 3.5
  dimension "d83" = 1
  constraint parallel L2 L4
  constraint perpendicular L3 L5
  constraint perpendicular L5 L6
  constraint perpendicular L4 L7
  constraint coincident P0 L4
  constraint coincident P0 L14
  constraint tangent L4 A0
  constraint tangent L14 A0
  constraint tangent L14 A1
  constraint tangent L13 A1
  constraint equal A0 A1
  constraint coincident P1 L13
  constraint coincident P1 L4
  constraint tangent L13 A2
  constraint tangent L4 A2
  constraint equal A0 A2
  constraint coincident P2 L12
  constraint coincident P2 L7
  constraint tangent L12 A3
  constraint tangent L7 A3
  constraint equal A0 A3
  constraint coincident P3 L7
  constraint coincident P3 L11
  constraint tangent L7 A4
  constraint tangent L11 A4
  constraint equal A0 A4
  constraint tangent L11 A5
  constraint tangent L12 A5
  constraint equal A0 A5
  constraint tangent L10 A6
  constraint tangent L9 A6
  constraint equal A0 A6
  constraint tangent L10 A7
  constraint tangent L5 A7
  constraint equal A0 A7
  constraint tangent L5 A8
  constraint tangent L9 A8
  constraint equal A0 A8
  constraint tangent L16 A9
  constraint tangent L6 A9
  constraint equal A0 A9
  constraint tangent L6 A10
  constraint tangent L15 A10
  constraint equal A0 A10
  constraint tangent L15 A11
  constraint tangent L16 A11
  constraint equal A0 A11
  measures "d75" distance of P0 P1
  measures "d76" distance of P2 P3
  measures "d77" distance of L1 P1
  measures "d78" distance of P2 L8
  measures "d79" distance of L2 L4
  measures "d80" distance of L0 L5
  measures "d81" distance of L1 L7
  measures "d82" distance of L3 L6
  measures "d83" radius of A0
extrude "Extrude6" cut sketch "Sketch10" against normal blind 2 contours L4 L13 L14 A0 A1 A2 | L5 L9 L10 A6 A7 A8 | L6 L15 L16 A9 A10 A11 | L7 L11 L12 A3 A4 A5
extrude "Extrude7" add 1 faces at (8.5, 16.6833, 0) along direction (0, 0, -1) blind 0.25
extrude "Extrude8" add 2 faces at (41, 10.6667, -0.0833) (41, 27.6732, 3.691) along direction (1, 0, 0) blind 20
sketch "Sketch12" plane through (0, 0, 6.5) normal (0, 0, 1) x (-1, 0, 0)
  arc A0 (-19, 41) -> (-21, 39) centre (-19, 39) ccw
  arc A1 (-23, 37) -> (-21, 39) centre (-23, 39) ccw
  line L0 (-23, 37) -> (-36, 37)
  arc A2 (-36, 37) -> (-41, 32) centre (-36, 32) ccw
  line L1 (-41, 32) -> (-61, 32)
  line L2 (-61, 32) -> (-61, 19.05)
  line L3 (-61, 19.05) -> (41, 19.05)
  line L4 (41, 19.05) -> (41, 32)
  arc A3 (41, 32) -> (36, 37) centre (36, 32) ccw
  line L5 (36, 37) -> (23, 37)
  arc A4 (21, 39) -> (23, 37) centre (23, 39) ccw
  arc A5 (21, 39) -> (19, 41) centre (19, 39) ccw
  line L6 (19, 41) -> (-19, 41)
  circle A6 centre (-34, 30) radius 5
  circle A7 centre (34, 30) radius 5
  circle A8 centre (10, 34.75) radius 2.5
  circle A9 centre (-10, 34.75) radius 2.5
  line L7 (-27.5, 24.05) -> (-27.5, 27.05)
  arc A10 (-25.5, 29.05) -> (-27.5, 27.05) centre (-25.5, 27.05) ccw
  line L8 (-25.5, 29.05) -> (25.5, 29.05)
  arc A11 (27.5, 27.05) -> (25.5, 29.05) centre (25.5, 27.05) ccw
  line L9 (27.5, 27.05) -> (27.5, 24.05)
  arc A12 (25.5, 22.05) -> (27.5, 24.05) centre (25.5, 24.05) ccw
  line L10 (25.5, 22.05) -> (-25.5, 22.05)
  arc A13 (-27.5, 24.05) -> (-25.5, 22.05) centre (-25.5, 24.05) ccw
  line L11 (-61, 32) -> (-41, 32)
  line L12 (-41, 32) -> (-41, 21.05)
  line L13 (-41, 21.05) -> (-61, 21.05)
  line L14 (-61, 21.05) -> (-61, 32)
  line L15 (-61, -32) -> (-41, -32)
  line L16 (-41, -32) -> (-41, -21.05)
  line L17 (-41, -21.05) -> (-61, -21.05)
  line L18 (-61, -21.05) -> (-61, -32)
  line L19 (41, -19.05) -> (-61, -19.05)
  dimension "d90" = 2
  dimension "d91" = 20
  dimension "d92" = 2
  dimension "d93" = 20
  dimension "d94" = 64
  constraint horizontal L11
  constraint vertical L12
  constraint horizontal L13
  constraint vertical L14
  constraint coincident L1.end L2.start
  constraint horizontal L15
  constraint vertical L16
  constraint horizontal L17
  constraint vertical L18
  constraint vertical L1.end L15.start
  measures "d90" distance of L3 L13
  measures "d91" distance of L12 L14
  measures "d92" distance of L17 L19
  measures "d93" distance of L16 L18
  measures "d94" distance of L11 L15
extrude "Extrude9" cut sketch "Sketch12" against normal blind 7 contours L1 L2 L11 L12 L13 L14 | L15 L16 L17 L18
fillet "Fillet4" radius 5 2 edges at (41, 21.05, 3.125) (41, -21.05, 3.125)
fillet "Fillet5" radius 1.5 2 edges at (61, 21.05, 3.125) (61, -21.05, 3.125)
sketch "Sketch14" plane through (0, 0, 2) normal (0, 0, 1) x (-1, 0, 0)
  line L0 (37.5, 10.6064) -> (37.5, -10.6064)
  arc A0 (36.1798, -11.5537) -> (37.5, -10.6064) centre (36.5, -10.6064) ccw
  line L1 (36.1798, -11.5537) -> (4.8025, -0.9473)
  arc A1 (4.8025, 0.9473) -> (4.8025, -0.9473) centre (5.1228, 0) ccw
  line L2 (4.8025, 0.9473) -> (36.1798, 11.5537)
  arc A2 (37.5, 10.6064) -> (36.1798, 11.5537) centre (36.5, 10.6064) ccw
  line L3 (30.154, 12.0513) -> (0.3162, 2.1054)
  arc A3 (-0.3162, 2.1054) -> (0.3162, 2.1054) centre (0, 3.0541) ccw
  line L4 (-0.3162, 2.1054) -> (-30.154, 12.0513)
  arc A4 (-29.8377, 14) -> (-30.154, 12.0513) centre (-29.8377, 13) ccw
  line L5 (-29.8377, 14) -> (29.8377, 14)
  arc A5 (30.154, 12.0513) -> (29.8377, 14) centre (29.8377, 13) ccw
  line L6 (-30.154, -12.0513) -> (-0.3162, -2.1054)
  arc A6 (0.3162, -2.1054) -> (-0.3162, -2.1054) centre (0, -3.0541) ccw
  line L7 (0.3162, -2.1054) -> (30.154, -12.0513)
  arc A7 (29.8377, -14) -> (30.154, -12.0513) centre (29.8377, -13) ccw
  line L8 (29.8377, -14) -> (-29.8377, -14)
  arc A8 (-30.154, -12.0513) -> (-29.8377, -14) centre (-29.8377, -13) ccw
  line L9 (-4.8025, -0.9473) -> (-36.1798, -11.5537)
  arc A9 (-37.5, -10.6064) -> (-36.1798, -11.5537) centre (-36.5, -10.6064) ccw
  line L10 (-37.5, -10.6064) -> (-37.5, 10.6064)
  arc A10 (-36.1798, 11.5537) -> (-37.5, 10.6064) centre (-36.5, 10.6064) ccw
  line L11 (-36.1798, 11.5537) -> (-4.8025, 0.9473)
  arc A11 (-4.8025, -0.9473) -> (-4.8025, 0.9473) centre (-5.1228, 0) ccw
  line L12 (41, 16.05) -> (-61, 16.05)
  line L13 (-61, 16.05) -> (-61, -16.05)
  line L14 (-61, -16.05) -> (41, -16.05)
  line L15 (41, -16.05) -> (41, 16.05)
  line L16 (-57.5, 10.5218) -> (-57.5, -10.5218)
  line L17 (-41, 10.5218) -> (-41, -10.5218)
  line L18 (-41.94, -10.7593) -> (-47.2368, -0.9503)
  line L19 (-47.2368, 0.9503) -> (-41.94, 10.7593)
  line L20 (-56.56, 10.7593) -> (-51.2632, 0.9503)
  line L21 (-51.2632, -0.9503) -> (-56.56, -10.7593)
  line L22 (-55.0268, 14) -> (-43.4732, 14)
  line L23 (-42.6049, 12.5039) -> (-48.3818, 2.3944)
  line L24 (-50.1182, 2.3944) -> (-55.8951, 12.5039)
  line L25 (-55.8951, -12.5039) -> (-50.1182, -2.3944)
  line L26 (-48.3818, -2.3944) -> (-42.6049, -12.5039)
  line L27 (-43.4732, -14) -> (-55.0268, -14)
  arc A12 (-55.0268, 14) -> (-55.8951, 12.5039) centre (-55.0268, 13) ccw
  arc A13 (-42.6049, 12.5039) -> (-43.4732, 14) centre (-43.4732, 13) ccw
  arc A14 (-55.8951, -12.5039) -> (-55.0268, -14) centre (-55.0268, -13) ccw
  arc A15 (-43.4732, -14) -> (-42.6049, -12.5039) centre (-43.4732, -13) ccw
  arc A16 (-48.3818, -2.3944) -> (-50.1182, -2.3944) centre (-49.25, -2.8906) ccw
  arc A17 (-50.1182, 2.3944) -> (-48.3818, 2.3944) centre (-49.25, 2.8906) ccw
  arc A18 (-41, 10.5218) -> (-41.94, 10.7593) centre (-41.5, 10.5218) ccw
  arc A19 (-41.94, -10.7593) -> (-41, -10.5218) centre (-41.5, -10.5218) ccw
  arc A20 (-57.5, -10.5218) -> (-56.56, -10.7593) centre (-57, -10.5218) ccw
  arc A21 (-51.2632, -0.9503) -> (-51.2632, 0.9503) centre (-53.023, 0) ccw
  arc A22 (-47.2368, 0.9503) -> (-47.2368, -0.9503) centre (-45.477, 0) ccw
  arc A23 (-56.56, 10.7593) -> (-57.5, 10.5218) centre (-57, 10.5218) ccw
  point P0 (-57.5, 12.5)
  point P1 (-57.5, -12.5)
  point P2 (-47.75, 0)
  point P3 (-50.75, 0)
  point P4 (-49.25, 0.875)
  point P5 (-56.75, -14)
  point P6 (-49.25, -0.875)
  point P7 (-41.75, -14)
  dimension "d106" = 3.5
  dimension "d107" = 3.5
  dimension "d108" = 2.05
  dimension "d109" = 2.05
  dimension "d110" = 25
  dimension "d111" = 12.5
  dimension "d112" = 15
  dimension "d113" = 0.75
  dimension "d114" = 3
  dimension "d115" = 1.75
  dimension "d116" = 1.5
  dimension "d117" = 0.875
  dimension "d118" = 8.25
  dimension "d119" = 1
  dimension "d120" = 0.5
  dimension "d121" = 2
  dimension "d122" = 0.5
  constraint vertical L16
  constraint perpendicular L12 L17
  constraint perpendicular L16 L22
  constraint horizontal P2 P3
  constraint vertical P4 P6
  constraint horizontal origin P2
  constraint tangent L24 A12
  constraint tangent L22 A12
  constraint tangent L22 A13
  constraint tangent L23 A13
  constraint equal A12 A13
  constraint coincident P5 L25
  constraint coincident P5 L27
  constraint tangent L25 A14
  constraint tangent L27 A14
  constraint equal A12 A14
  constraint coincident P7 L27
  constraint coincident P7 L26
  constraint tangent L27 A15
  constraint tangent L26 A15
  constraint equal A12 A15
  constraint coincident P6 L26
  constraint coincident P6 L25
  constraint tangent L26 A16
  constraint tangent L25 A16
  constraint equal A12 A16
  constraint coincident P4 L24
  constraint coincident P4 L23
  constraint tangent L24 A17
  constraint tangent L23 A17
  constraint equal A12 A17
  constraint tangent L19 A18
  constraint tangent L17 A18
  constraint tangent L17 A19
  constraint tangent L18 A19
  constraint equal A18 A19
  constraint coincident P1 L21
  constraint coincident P1 L16
  constraint tangent L21 A20
  constraint tangent L16 A20
  constraint equal A18 A20
  constraint coincident P3 L20
  constraint coincident P3 L21
  constraint tangent L20 A21
  constraint tangent L21 A21
  constraint coincident P2 L18
  constraint coincident P2 L19
  constraint tangent L18 A22
  constraint tangent L19 A22
  constraint equal A21 A22
  constraint coincident P0 L16
  constraint coincident P0 L20
  constraint tangent L16 A23
  constraint tangent L20 A23
  measures "d106" distance of L13 L16
  measures "d107" distance of L10 L17
  measures "d108" distance of L12 L22
  measures "d109" distance of L14 L27
  measures "d110" distance of P0 P1
  measures "d111" vertical distance of origin P0
  measures "d112" distance of P5 P7
  measures "d113" horizontal distance of P1 P5
  measures "d114" distance of P2 P3
  measures "d115" distance of P4 P6
  measures "d116" horizontal distance of P3 P4
  measures "d117" vertical distance of P2 P6
  measures "d118" distance of L17 P4
  measures "d119" radius of A12
  measures "d120" radius of A18
  measures "d121" radius of A21
  measures "d122" radius of A23
extrude "Extrude11" cut sketch "Sketch14" against normal blind 3 contours L16 L20 L21 A20 A21 A23 | L17 L18 L19 A18 A19 A22 | L22 L23 L24 A12 A13 A17 | L25 L26 L27 A14 A15 A16
equation "d3 = ( 82 / 2 ) * 1 mm"
equation "d4 = ( 82 / 2 ) * 1 mm"
equation "d9 = ( ( 82 - 68 ) / 2 ) * 1 mm"
equation "d10 = ( ( 82 - 60 ) / 2 ) * 1 mm"
equation "d17 = ( 38.1 / 2 ) * 1 mm"
equation "d26 = ( ( 82 - 20 ) / 2 ) * 1 mm"
equation "d34 = ( ( 82 - 55 ) / 2 ) * 1 mm"
equation "d37 = ( ( 82 - 55 ) / 2 ) * 1 mm"
equation "d77 = ( ( 82 - 72 ) / 2 ) * 1 mm"
equation "d78 = ( ( 38.1 - 24 ) / 2 ) * 1 mm"
equation "d113 = ( ( 16.5 - 15 ) / 2 ) * 1 mm"
equation "d117 = ( 1.75 / 2 ) * 1 mm"
equation "d118 = ( 16.5 / 2 ) * 1 mm"

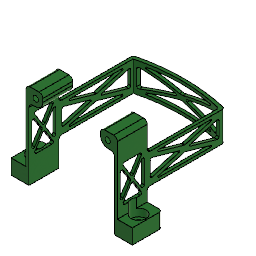
design "TM Back Holder"
Autodesk Fusion 360 part; units mm, degrees
sketch "Sketch1" plane through (0, 0, 0) normal (0, 0, 1) x (1, 0, 0)
  line L0 (-30.55, 69.6) -> (-28.55, 69.6)
  line L1 (-28.55, 69.6) -> (-28.55, 0)
  line L2 (-28.55, 0) -> (-30.55, 0)
  line L3 (-30.55, 0) -> (-30.55, 69.6)
  line L4 (28.55, 69.6) -> (30.55, 69.6)
  line L5 (30.55, 69.6) -> (30.55, 0)
  line L6 (30.55, 0) -> (28.55, 0)
  line L7 (28.55, 0) -> (28.55, 69.6)
  dimension "d1" = 69.6
  dimension "d2" = 69.6
  dimension "d3" = 2
  dimension "d4" = 2
  dimension "d5" = 57.1
  dimension "d6" = 28.55
  constraint horizontal L0
  constraint vertical L1
  constraint horizontal L2
  constraint vertical L3
  constraint horizontal L4
  constraint vertical L5
  constraint horizontal L6
  constraint vertical L7
  constraint horizontal L0.start L4.start
  constraint horizontal origin L1.end
  measures "d1" distance of L0 L2
  measures "d2" distance of L4 L6
  measures "d3" distance of L1 L3
  measures "d4" distance of L5 L7
  measures "d5" distance of L1 L7
  measures "d6" distance of origin L7
extrude "Extrude1" add sketch "Sketch1" along normal blind 20 makes body 1 at (-28.55, 46.4, 6.6667) makes body 2 at (30.55, 46.4, 6.6667)
sketch "Sketch3" plane through (0, 0, 20) normal (0, 0, 1) x (-1, 0, 0)
  line L0 (-28.55, 0) -> (-30.55, 0)
  line L1 (-30.55, 0) -> (-30.55, -69.6)
  line L2 (-30.55, -69.6) -> (-28.55, -69.6)
  line L3 (-28.55, -69.6) -> (-28.55, 0)
  arc A0 (-28.55, -69.6) -> (28.55, -69.6) centre (0, 38.699) ccw
  arc A1 (-30.55, -71.6) -> (30.55, -71.6) centre (0, 52.672) ccw
  line L4 (30.55, -71.6) -> (30.55, -69.6)
  line L5 (-30.55, -71.6) -> (-30.55, -69.6)
  line L6 (-28.55, -69.6) -> (-30.55, -69.6)
  line L7 (28.55, -69.6) -> (30.55, -69.6)
  point P0 (-28.55, -69.6)
  point P1 (28.55, -69.6)
  point P2 (0, -73.3)
  point P3 (0, -75.3)
  point P4 (30.55, -71.6)
  point P5 (-30.55, -71.6)
  point P6 (30.55, -69.6)
  dimension "d9" = 3.7
  dimension "d10" = 2
  dimension "d11" = 2
  dimension "d12" = 2
  constraint coincident P0 L2.end
  constraint coincident P2 A0
  constraint coincident P1 A0.end
  constraint vertical origin P2
  constraint vertical P2 P3
  constraint vertical L1.end P5
  constraint vertical P4 P6
  constraint coincident P3 A1
  constraint coincident P5 A1.start
  constraint coincident P4 A1.end
  constraint coincident P6 L4.end
  constraint coincident L1.end L2.start
  measures "d9" vertical distance of P0 P2
  measures "d10" distance of P2 P3
  measures "d11" distance of P4 P6
  measures "d12" distance of L1.end P5
extrude "Extrude2" add sketch "Sketch3" against normal blind 20 contours L2 A0 A1 L4 L5 L6 L7 bodies 1 2
sketch "Sketch4" plane through (30.55, 0, 0) normal (1, 0, 0) x (0, 1, 0)
  line L0 (0, 0) -> (71.6, 0)
  line L1 (71.6, 0) -> (71.6, 20)
  line L2 (71.6, 20) -> (0, 20)
  line L3 (0, 20) -> (0, 0)
  line L4 (0, 0) -> (20, 0)
  line L5 (20, 0) -> (20, -4)
  line L6 (20, -4) -> (0, -4)
  line L7 (0, -4) -> (0, 0)
  dimension "d15" = 4
  dimension "d16" = 20
  constraint horizontal L4
  constraint vertical L5
  constraint horizontal L6
  constraint vertical L7
  constraint coincident L0.start L3.end
  measures "d15" distance of L4 L6
  measures "d16" distance of L5 L7
extrude "Extrude3" add sketch "Sketch4" against normal blind 2 contours L0 L4 L5 L6 L7 bodies 1
sketch "Sketch5" plane through (-30.55, 0, 0) normal (-1, 0, 0) x (0, -1, 0)
  line L0 (-71.6, 0) -> (0, 0)
  line L1 (0, 0) -> (0, 20)
  line L2 (0, 20) -> (-71.6, 20)
  line L3 (-71.6, 20) -> (-71.6, 0)
  line L4 (0, 0) -> (-20, 0)
  line L5 (-20, 0) -> (-20, -4)
  line L6 (-20, -4) -> (0, -4)
  line L7 (0, -4) -> (0, 0)
  dimension "d19" = 4
  dimension "d20" = 20
  constraint horizontal L4
  constraint vertical L5
  constraint horizontal L6
  constraint vertical L7
  constraint coincident L0.end L1.start
  measures "d19" distance of L4 L6
  measures "d20" distance of L5 L7
extrude "Extrude4" add sketch "Sketch5" against normal blind 2 contours L0 L4 L5 L6 L7 bodies 1
fillet "Fillet2" radius 2 4 edges at (30.55, 71.6, 10) (-30.55, 71.6, 10) (29.55, 20, 0) (-29.55, 20, 0) on bodies 1